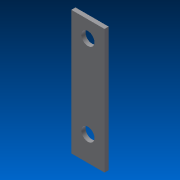
# Autodesk Inventor part: SpacerBasket
Saved by Autodesk Inventor 2013 (Build 170138000, 138)
## iProperties
Created: 2013-08-02
Part Number: SpacerBasket
Material: Generic
Document SubType Name: Modeling
Designer: nowireless
Density: 1 g/cm^3
Author: nowireless
Autodesk Inventor part; units mm, degrees
ref_plane "YZ Plane" through (0, 0, 0) normal (1, 0, 0) x (0, 1, 0)
ref_plane "XZ Plane" through (0, 0, 0) normal (0, 1, 0) x (-1, 0, 0)
ref_plane "XY Plane" through (0, 0, 0) normal (0, 0, 1) x (1, 0, 0)
sketch "Sketch1" plane through (0, 0, 0) normal (0, 0, 1) x (1, 0, 0)
  line L0 (0, 0) -> (12.7, 0)
  line L1 (12.7, 0) -> (12.7, 47.625)
  line L2 (12.7, 47.625) -> (0, 47.625)
  line L3 (0, 47.625) -> (0, 0)
  dimension "d0" = 47.625
  dimension "d1" = 12.7
  constraints: 8 end point, 2 parallel, 1 horizontal, 1 perpendicular
  measures "d0" distance of L2.end L0.start
  measures "d1" distance of L0.start L0.end
extrude "Extrusion1" add sketch "Sketch1" along normal blind 1.5875
sketch "Sketch2" plane through (0, 0, 1.5875) normal (0, 0, 1) x (1, 0, 0)
  line L0 (12.7, 0) -> (12.7, 47.625) projected
  line L1 (12.7, 47.625) -> (0, 47.625) projected
  line L2 (0, 47.625) -> (0, 0) projected
  point P0 (6.35, 41.275)
  point P1 (6.35, 9.525)
  dimension "d4" = 31.75
  dimension "d6" = 6.35
  dimension "d7" = 6.35
  dimension "d8" = 6.35
  measures "d4" distance of point (6.35, 41.275) point (6.35, 9.525)
  measures "d6" distance from line of point (6.35, 41.275) L1
  measures "d7" distance from line of L0 point (6.35, 41.275)
  measures "d8" distance from line of L2 point (6.35, 9.525)
hole "Hole1" at (6.35, 41.275, 1.5875) at (6.35, 9.525, 1.5875) direction (0, 0, -1) diameter 5 depth 25.4 tip angle 118
body "Solid1"
